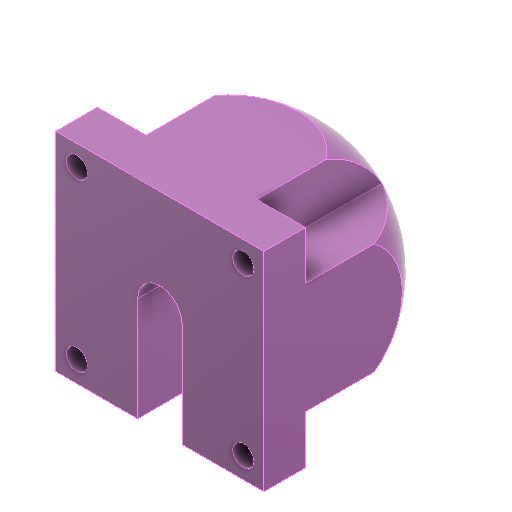
# Autodesk Inventor part: sujecion_cable_2
Saved by Autodesk Inventor 2026.1 (Build 301233000, 233)
## iProperties
Created: 2025-10-01
Part Number: sujecion_cable_2
Material: Genérico
Document SubType Name: Modeling
Designer: gianm
Density: 1 g/cm^3
Appearance: Suave - Púrpura
Author: gianm
Autodesk Inventor part; units mm, degrees
ref_plane "YZ Plane" through (0, 0, 0) normal (1, 0, 0) x (0, 1, 0)
ref_plane "XZ Plane" through (0, 0, 0) normal (0, 1, 0) x (-1, 0, 0)
sketch "Boceto1" plane through (0, 0, 0) normal (0, 0, 1) x (1, 0, 0)
  line L0 (-7.5, -7.5) -> (7.5, -7.5)
  line L1 (7.5, -7.5) -> (7.5, 7.5)
  line L2 (7.5, 7.5) -> (-7.5, 7.5)
  line L3 (-7.5, 7.5) -> (-7.5, -7.5)
  line L4 (-7.5, -7.5) -> (7.5, 7.5) construction
  line L5 (7.5, -7.5) -> (-7.5, 7.5) construction
  point P0 (0, 0)
  dimension "d0" = 15
  constraints: 12 end point, 2 midpoint, 2 parallel, 1 horizontal, 1 perpendicular
  measures "d0" distance of L1.end L2.end
extrude "Extrusión1" add sketch "Boceto1" against normal blind 5
ref_plane "Plano de trabajo1" through (0, -7.5, 0) normal (1, 0, 0) x (0, 0, -1)
sketch "Boceto2" plane through (0, -7.5, 0) normal (1, 0, 0) x (0, 0, -1)
  line L0 (5, 15) -> (5, 0) projected
  arc A0 (14, 7.5) -> (5, 16.5) centre (5, 7.5) ccw
  line L1 (5, 7.5) -> (14, 7.5)
  line L2 (5, 7.5) -> (5, 16.5)
  point P0 (0, 7.5)
  dimension "d5" = 9
  constraints: 4 end point, 2 point on circle, 1 centre point, 1 horizontal, 1 midpoint, 1 vertical
  measures "d5" radius of A0
revolve "Revolución1" add sketch "Boceto2" angle 360 about axis through (0, 0, -5) along (0, 0, -1)
sketch "Boceto3" plane through (0, 0, 0) normal (0, 0, 1) x (1, 0, 0)
  line L0 (-7.5, 7.5) -> (-7.5, -7.5) projected
  line L1 (-7.5, 7.5) -> (7.5, 7.5)
  line L2 (7.5, 7.5) -> (7.5, -7.5)
  line L3 (7.5, -7.5) -> (-7.5, -7.5)
  line L4 (-7.5, -7.5) -> (-7.5, 7.5)
  circle A0 centre (0, 0) radius 9
  arc A1 (-4.9749, -7.5) -> (4.9749, -7.5) centre (0, 0) ccw projected
  line L5 (-7.5, -7.5) -> (7.5, -7.5) projected
  line L6 (7.5, -7.5) -> (7.5, 7.5) projected
  line L7 (-7.5, 7.5) -> (-4, 7.5)
  line L8 (-4, 7.5) -> (-4, 4)
  line L9 (-4, 4) -> (-7.5, 4)
  line L10 (-7.5, 4) -> (-7.5, 7.5)
  line L11 (-7.5, -7.5) -> (-7.5, -4)
  line L12 (-7.5, -4) -> (-4, -4)
  line L13 (-4, -4) -> (-4, -7.5)
  line L14 (-4, -7.5) -> (-7.5, -7.5)
  line L15 (7.5, -7.5) -> (4, -7.5)
  line L16 (4, -7.5) -> (4, -4)
  line L17 (4, -4) -> (7.5, -4)
  line L18 (7.5, -4) -> (7.5, -7.5)
  line L19 (7.5, 7.5) -> (7.5, 4)
  line L20 (7.5, 4) -> (4, 4)
  line L21 (4, 4) -> (4, 7.5)
  line L22 (4, 7.5) -> (7.5, 7.5)
  point P0 (-7.5, -7.5)
  point P1 (7.5, -4.9749)
  point P2 (7.5, 4.9749)
  point P3 (7.5, -4)
  point P4 (4, -7.5)
  point P5 (4, 7.5)
  point P6 (7.5, 4)
  dimension "d9" = 3.5
  dimension "d12" = 360
  constraints: 40 end point, 4 parallel, 3 coincident, 3 perpendicular, 2 collinear, 2 horizontal, 1 centre point, 1 concentric, 35 other
  measures "d9" distance of L7.end L8.end
extrude "Extrusión2" cut sketch "Boceto3" against normal up to next contours L0 A0 | L0 A0 L1 L8 L9 | L12 L13 L3 A0 L0 | L0 L1 A0 | A0 L3 L0 | A0 L1 | L3 A0 | A0 L2 L20 L21 L1 | L1 L2 A0 | A0 L2 L3 | L3 L16 L17 L2 A0 | A0 L2
sketch "Boceto4" plane through (0, 0, 0) normal (0, 0, 1) x (1, 0, 0)
  line L0 (-7.5, -7.5) -> (7.5, -7.5)
  line L1 (7.5, -7.5) -> (7.5, 7.5)
  line L2 (7.5, 7.5) -> (-7.5, 7.5)
  line L3 (-7.5, 7.5) -> (-7.5, -7.5)
  line L4 (-7.5, -7.5) -> (7.5, 7.5) construction
  line L5 (7.5, -7.5) -> (-7.5, 7.5) construction
  line L6 (4, 7.5) -> (-4, 7.5) projected
  line L7 (7.5, -4) -> (7.5, 4) projected
  point P0 (0, 0)
  constraints: 12 end point, 2 collinear, 2 midpoint, 2 parallel, 1 horizontal, 1 perpendicular
extrude "Extrusión3" add sketch "Boceto4" against normal blind 3
sketch "Boceto5" plane through (0, 0, 0) normal (0, 0, 1) x (1, 0, 0)
  circle A0 centre (-6, -6) radius 0.75
  circle A1 centre (6, -6) radius 0.75
  circle A2 centre (6, 6) radius 0.75
  circle A3 centre (-6, 6) radius 0.75
  circle A4 centre (0, 0) radius 1.6
  dimension "d16" = 1.5
  dimension "d19" = 360
  dimension "d25" = 3.2
  constraints: 5 centre point, 1 coincident, 9 other
  measures "d16" diameter of A0
  measures "d25" diameter of A4
extrude "Extrusión4" cut sketch "Boceto5" against normal up to next
sketch "Boceto6" plane through (-7.5, -7.5, 0) normal (0, -1, 0) x (1, 0, 0)
  line L0 (5.9, 7) -> (5.9, -7)
  line L1 (5.9, -7) -> (9.1, -7)
  line L2 (9.1, -7) -> (9.1, 7)
  line L3 (9.1, 7) -> (5.9, 7)
  line L4 (5.9, 7) -> (9.1, -7) construction
  line L5 (5.9, -7) -> (9.1, 7) construction
  point P0 (7.5, 0)
  point P1 (7.5, 0)
  dimension "d26" = 3.2
  dimension "d27" = 7
  constraints: 12 end point, 3 midpoint, 2 parallel, 1 perpendicular, 1 vertical
  measures "d26" distance of L0.end L1.end
  measures "d27" distance from line of point (7.5, 0) L1
extrude "Extrusión5" cut sketch "Boceto6" against normal blind 7.5
